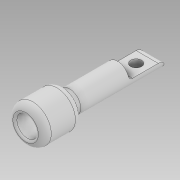
# Autodesk Inventor part: 3103a_Bulb Arm_BulbHolder_V2_B
Saved by Autodesk Inventor 2020 (Build 240168000, 168)
## iProperties
Created: 2020-09-10
Part Number: 3103a_Bulb Arm_BulbHolder_V2_B
Material: Generic
Document SubType Name: Modeling
Designer: Eli Mattingly
Density: 1 g/cm^3
Appearance: Default
Author: Eli Mattingly
Autodesk Inventor part; units mm, degrees
ref_plane "YZ Plane" through (0, 0, 0) normal (1, 0, 0) x (0, 1, 0)
ref_plane "XZ Plane" through (0, 0, 0) normal (0, 1, 0) x (-1, 0, 0)
ref_plane "XY Plane" through (0, 0, 0) normal (0, 0, 1) x (1, 0, 0)
sketch "Sketch1" plane through (0, 0, 0) normal (0, 0, 1) x (1, 0, 0)
  circle A0 centre (0, 0) radius 3
  dimension "d0" = 6
  constraints: 1 centre point, 1 coincident
  measures "d0" diameter of A0
extrude "Extrusion1" add sketch "Sketch1" along normal blind 25
sketch "Sketch2" plane through (0, 0, 0) normal (0, 0, -1) x (-1, 0, 0)
  circle A0 centre (0, 0) radius 3 projected
  line L0 (-3, 0) -> (3, 0)
  constraints: 2 end point, 2 point on circle, 1 horizontal
extrude "Extrusion2" add sketch "Sketch2" along normal blind 10 contours A0 L0 picked at (-0.8855, -0.4647)
fillet "Fillet1" radius 2 1 edges at (0, 0, -10)
fillet "Fillet2" radius 1 1 edges at (0, 0, 0)
sketch "Sketch7" plane through (0, 0, 25) normal (0, 0, 1) x (1, 0, 0)
  circle A0 centre (0, 0) radius 3 projected
  circle A1 centre (0, 0) radius 2.85
  dimension "d25" = 5.7
  constraints: 1 centre point, 1 coincident
  measures "d25" diameter of A1
extrude "Extrusion7" cut sketch "Sketch7" against normal blind 10 contours A1
sketch "Sketch8" plane through (0, 0, 25) normal (0, 0, 1) x (1, 0, 0)
  circle A0 centre (0, 0) radius 3 projected
  circle A1 centre (0, 0) radius 5
  dimension "d28" = 10
  constraints: 1 centre point, 1 coincident
  measures "d28" diameter of A1
extrude "Extrusion8" add sketch "Sketch8" against normal blind 10
fillet "Fillet7" radius 2 3 edges at (-3, 0, 15) (-5, 0, 15) (-5, 0, 25)
fillet "Fillet8" radius 0.5 1 edges at (-2.85, 0, 25)
sketch "Sketch9" plane through (-3, 0, -8) normal (0, 1, 0) x (1, 0, 0)
  line L0 (3, -8) -> (3, -3)
  circle A0 centre (3, -3) radius 1.5
  dimension "d33" = 5
  dimension "d34" = 3
  constraints: 2 end point, 1 centre point, 1 coincident, 1 vertical
  measures "d33" distance of L0.start L0.end
  measures "d34" diameter of A0
extrude "Extrusion9" cut sketch "Sketch9" against normal blind 10
body "Solid1"
